A3 (Autodesk Fusion 360 design; units mm, degrees)
Autodesk Fusion 360 part; units mm, degrees
sketch "Sketch" plane through (0, 0, 0) normal (0, 0, 1) x (-1, 0, 0)
  line L0 (-88, 67) -> (0, 67)
  line L1 (0, 67) -> (0, 0)
  line L2 (0, 0) -> (-88, 0)
  line L3 (-88, 0) -> (-88, 67)
  circle A0 centre (-19, 31) radius 5
  circle A1 centre (-69, 31) radius 5
  line L4 (-44, 67) -> (-30.7145, 80.5829) construction
  arc A2 (-30.7145, 80.5829) -> (-57.5829, 80.2855) centre (-44, 67) ccw
  line L5 (-44, 67) -> (-57.5829, 80.2855) construction
  line L6 (-44, 67) -> (-30.7145, 80.5829) construction
  line L7 (-30.7145, 80.5829) -> (0, 50.5408)
  line L8 (-57.5829, 80.2855) -> (-88, 49.1876)
  circle A3 centre (-13, 45.0716) radius 13
  circle A4 centre (-75, 43.8869) radius 13
  line L9 (0, 0) -> (-88, 0)
  line L10 (-63, 3) -> (-25, 3)
  circle A5 centre (-22, 3) radius 3
  circle A6 centre (-66, 3) radius 3
  line L11 (-25, 3) -> (-63, 3)
  line L12 (0, -13) -> (0, 0)
  line L13 (-88, -13) -> (0, -13)
  line L14 (0, 0) -> (-88, 0)
  line L15 (-88, 0) -> (-88, -13)
  line L16 (-44, 67) -> (-39, 67)
  line L17 (-39, 67) -> (-49, 67)
  line L18 (-39, 3) -> (-39, 67)
  line L19 (-49, 67) -> (-49, 3)
  line L20 (-49, 3) -> (-39, 3)
  line L21 (-49, 3) -> (-49, 7)
  line L22 (-39, 3) -> (-49, 3)
  line L23 (-39, 7) -> (-39, 3)
  line L24 (-49, 7) -> (-39, 7)
  circle A7 centre (-44, -19) radius 9.5
  circle A8 centre (-44, -19) radius 19
  line L25 (-44, -13) -> (-44, -19)
  line L26 (0, -13) -> (-44, -13)
  circle A9 centre (-19, -19) radius 6
  line L27 (-44, -13) -> (-44, -19)
  line L28 (-88, -13) -> (-44, -13)
  circle A10 centre (-69, -19) radius 6
  point P0 (-70.5776, 67)
  point P1 (-16.8276, 67)
  dimension "d1" = 67
  dimension "d6" = 10
  dimension "d7" = 10
  dimension "d11" = 19
  dimension "d12" = 50
  dimension "d13" = 13
  dimension "d14" = 13
  dimension "d15" = 88
  dimension "d25" = 31
  dimension "d30" = 3
  dimension "d31" = 3
  dimension "d32" = 38
  dimension "d33" = 13
  dimension "d35" = 64
  dimension "d36" = 10
  dimension "d37" = 4
  dimension "d39" = 19
  dimension "d40" = 19
  dimension "d41" = 38
  dimension "d42" = 6
  dimension "d43" = 6
  constraint horizontal L0
  constraint horizontal L2
  constraint vertical L1
  constraint vertical L3
  constraint coincident L1.end L2.start
  constraint coincident L4.start A2.centre
  constraint coincident L1 L7.end
  constraint perpendicular L4 L7
  constraint coincident L3 L8.end
  constraint tangent A2 L8
  constraint tangent L7 A3
  constraint tangent L1 A3
  constraint tangent L8 A4
  constraint tangent L3 A4
  constraint horizontal L9
  constraint coincident L0 P0
  constraint coincident L8 P0
  constraint coincident L0 P1
  constraint coincident L7 P1
  constraint horizontal L10
  constraint tangent L9 A5
  constraint tangent L9 A6
  constraint parallel L10 L11
  constraint vertical L12
  constraint horizontal L13
  constraint vertical L15
  constraint horizontal L14
  constraint coincident L0 L16.end
  constraint horizontal L17
  constraint vertical L18
  constraint vertical L19
  constraint horizontal L20
  constraint vertical L21
  constraint horizontal L22
  constraint horizontal L24
  constraint vertical L23
  constraint concentric A7 A8
  constraint coincident A7.centre A8.centre
  constraint vertical L25
  constraint horizontal L26
  constraint tangent L26 A9
  constraint vertical L27
  constraint horizontal L28
  constraint tangent L28 A10
  measures "d1" distance of L0.end L1.end
  measures "d6" diameter of A0
  measures "d7" diameter of A1
  measures "d11" radius of A2
  measures "d12" distance of A0.centre A1.centre
  measures "d13" radius of A3
  measures "d14" radius of A4
  measures "d15" distance of L1.end L2.end
  measures "d25" vertical distance of A1.centre L2.end
  measures "d30" radius of A5
  measures "d31" radius of A6
  measures "d32" distance of L10.end L10.start
  measures "d33" distance of L1.end L12.start
  measures "d35" distance of L16.end L18.start
  measures "d36" distance of L16.end L17.end
  measures "d37" distance of L18.start L23.start
  measures "d39" diameter of A7
  measures "d40" distance of L14 A7.centre
  measures "d41" diameter of A8
  measures "d42" radius of A9
  measures "d43" radius of A10
extrude "Extrude2" add sketch "Sketch" along normal blind 10 contours L0 A2 L7 L8 L16 L17 | L0 L2 L3 A1 L8 A4 L9 L10 A6 L11 L14 L19 L21 | L0 L1 L2 A0 L7 A3 L9 L10 A5 L11 L14 L18 L23 | A1 A4 | A6 | A0 A3 | A5 picked at (-77.2796, 48.9706) picked at (-10.783, 49.7865)
extrude "Extrude3" add sketch "Sketch" along normal blind 40 contours L0 L16 L17 L18 L19 L24
chamfer "Chamfer1" distance 60 distance2 30 1 edges at (44, -67, 40) measured on face at (45.6667, -47, 40)
extrude "Extrude4" add sketch "Sketch" along normal blind 40 contours L10 L11 L18 L19 L20 L21 L22 L23 L24 | L2 L9 L10 A5 A6 L11 L14 L20 L22 | L2 L9 L13 L14 L15 A8 L28 | L2 L9 L12 L13 L14 A8 L26 | L13 A7 A8 L26 L28 | L13 A8 L28 A10 | A10 | L13 A7 A8 L26 L28 | L13 A8 L26 A9
extrude "Extrude5" cut sketch "Sketch" along normal blind 50 contours A10
